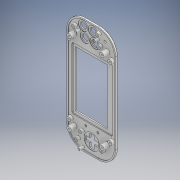
# Autodesk Inventor part: Partie Haute
Saved by Autodesk Inventor 2019 (Build 230136000, 136)
## iProperties
Created: 2018-06-04
Part Number: Partie Haute
Material: Plastique ABS
Document SubType Name: Modeling
Designer: dimercur
Mass: 33.4768 g
Surface Area: 274.719 cm^2
Volume: 31.5819 cm^3
Density: 1.06 g/cm^3
Appearance: Lisse - Blanc
Author: dimercur
Autodesk Inventor part; units mm, degrees
ref_plane "YZ Plane" through (0, 0, 0) normal (1, 0, 0) x (0, 1, 0)
ref_plane "XZ Plane" through (0, 0, 0) normal (0, 1, 0) x (-1, 0, 0)
ref_plane "XY Plane" through (0, 0, 0) normal (0, 0, 1) x (1, 0, 0)
sketch "Esquisse1" plane through (0, 0, 0) normal (0, 1, 0) x (-1, 0, 0)
  line L0 (42.5, 100) -> (-42.5, 100)
  line L1 (-42.5, 100) -> (-42.5, -100)
  line L2 (-42.5, -100) -> (42.5, -100)
  line L3 (42.5, -100) -> (42.5, 100)
  point P0 (0, 0)
  dimension "d0" = 200
  dimension "d1" = 85
  dimension "d2" = 42.5
  dimension "d3" = 100
  constraints: 8 end point, 2 parallel, 1 horizontal, 1 perpendicular
  measures "d0" distance of L2.end L0.start
  measures "d1" distance of L0.start L0.end
  measures "d2" horizontal distance of point (0, 0) L0.start
  measures "d3" vertical distance of point (0, 0) L0.start
extrude "Extrusion1" add sketch "Esquisse1" along normal blind 42
chamfer "Chanfrein1" distance 20 angle 60 1 edges at (0, 0, 100) measured on face at (-14.1667, 14, 100)
chamfer "Chanfrein2" distance 20 angle 60 1 edges at (0, 0, -100) measured on face at (14.1667, 14, -100)
fillet "Congé3" radius 30 4 edges at (-42.5, 31, 100) (42.5, 31, 100) (-42.5, 31, -100) (42.5, 31, -100)
fillet "Congé4" radius 15 14 edges at (0, 0, 65.359) (-33.7132, 14.9269, 91.2132) (-42.5, 1.3397, 67.6795) (33.7132, 14.9269, 91.2132) (42.5, 1.3397, 67.6795) (0, 20, 100) (-42.5, 0, 0) (42.5, 0, 0) (0, 0, -65.359) (33.7132, 14.9269, -91.2132) (42.5, 1.3397, -67.6795) (-33.7132, 14.9269, -91.2132) (-42.5, 1.3397, -67.6795) (0, 20, -100)
shell "Coque1" thickness 2.5 removed faces 1 at (-14.1667, 42, -23.3333)
sketch "Esquisse3" plane through (0, 42, 0) normal (0, 1, 0) x (1, 0, 0)
  arc A0 (42.5, 70) -> (12.5, 100) centre (12.5, 70) ccw projected
  line L0 (12.5, 100) -> (-12.5, 100) projected
  arc A1 (-12.5, 100) -> (-42.5, 70) centre (-12.5, 70) ccw projected
  line L1 (-42.5, 70) -> (-42.5, -70) projected
  arc A2 (-42.5, -70) -> (-12.5, -100) centre (-12.5, -70) ccw projected
  line L2 (-12.5, -100) -> (12.5, -100) projected
  arc A3 (12.5, -100) -> (42.5, -70) centre (12.5, -70) ccw projected
  line L3 (42.5, -70) -> (42.5, 70) projected
  point P0 (0, 0)
extrude "Extrusion2" add sketch "Esquisse3" along normal blind 2.5
sketch "Esquisse4" plane through (0, 44.5, 0) normal (0, 1, 0) x (1, 0, 0)
  line L0 (36.5, 54) -> (-34.5, 54)
  line L1 (-34.5, 54) -> (-34.5, -54)
  line L2 (-34.5, -54) -> (36.5, -54)
  line L3 (36.5, -54) -> (36.5, 54)
  line L4 (27.5, -67.5897) -> (-27.5, -67.5897) projected
  line L5 (42.5, -70) -> (42.5, 70) projected
  line L6 (-42.5, 70) -> (-42.5, -70) projected
  line L7 (12.5, 100) -> (-12.5, 100) projected
  line L8 (-12.5, -100) -> (12.5, -100) projected
  point P0 (0, 0)
  dimension "d19" = 108
  dimension "d20" = 71
  dimension "d21" = 36.5
  dimension "d22" = 54
  dimension "d154" = 85
  dimension "d155" = 46
  constraints: 8 end point, 2 parallel, 1 horizontal, 1 perpendicular
  measures "d19" distance of L2.end L0.start
  measures "d20" distance of L0.start L0.end
  measures "d21" horizontal distance of point (0, 0) L0.start
  measures "d22" vertical distance of point (0, 0) L0.start
  measures "d154" distance between parallel lines of L6 L5
  measures "d155" distance between parallel lines of L8 L2
extrude "Extrusion15" cut sketch "Esquisse4" against normal through all
sketch "Esquisse5" plane through (-40, 15, 61.3397) normal (1, 0, 0) x (0, 0, -1)
  line L0 (-48.6603, 26) -> (171.3397, 26)
  line L1 (171.3397, 26) -> (171.3397, -24)
  line L2 (171.3397, -24) -> (-48.6603, -24)
  line L3 (-48.6603, -24) -> (-48.6603, 26)
  line L4 (-36.1603, 27) -> (-8.6603, 27) projected
  line L5 (-38.6603, 29.5) -> (-38.6603, 13.6603) projected
  line L6 (161.3397, 13.6603) -> (161.3397, 29.5) projected
  point P0 (61.3397, -15)
  dimension "d47" = 1
  dimension "d48" = 220
  dimension "d50" = 200
  dimension "d51" = 10
  dimension "d52" = 50
  constraints: 8 end point, 2 parallel, 1 horizontal, 1 perpendicular
  measures "d47" distance between parallel lines of L4 L0
  measures "d48" distance between parallel lines of L1 L3
  measures "d50" distance between parallel lines of L6 L5
  measures "d51" distance between parallel lines of L5 L3
  measures "d52" distance between parallel lines of L0 L2
extrude "Extrusion4" cut sketch "Esquisse5" along normal through all both and the other way through all
sketch "Esquisse6" plane through (-12.5, 41, -100) normal (0, -1, 0) x (1, 0, 0)
  line L0 (-27.5, 170) -> (-27.5, 30) projected
  arc A0 (-27.5, 30) -> (0, 2.5) centre (0, 30) ccw projected
  line L1 (0, 2.5) -> (25, 2.5) projected
  arc A1 (25, 2.5) -> (52.5, 30) centre (25, 30) ccw projected
  line L2 (52.5, 30) -> (52.5, 170) projected
  arc A2 (52.5, 170) -> (25, 197.5) centre (25, 170) ccw projected
  line L3 (25, 197.5) -> (0, 197.5) projected
  arc A3 (0, 197.5) -> (-27.5, 170) centre (0, 170) ccw projected
  line L4 (-27.75, 30) -> (-27.75, 170)
  arc A4 (0, 197.75) -> (-27.75, 170) centre (0, 170) ccw
  line L5 (0, 197.75) -> (25, 197.75)
  arc A5 (52.75, 170) -> (25, 197.75) centre (25, 170) ccw
  line L6 (52.75, 170) -> (52.75, 30)
  arc A6 (25, 2.25) -> (52.75, 30) centre (25, 30) ccw
  line L7 (25, 2.25) -> (0, 2.25)
  arc A7 (-27.75, 30) -> (0, 2.25) centre (0, 30) ccw
  line L8 (-30, 30) -> (-30, 170) projected
  point P0 (12.5, 100)
  dimension "d55" = 2.5
  dimension "d56" = 0.25
  constraints: 8 end point, 8 point on circle, 4 centre point, 7 other
  measures "d55" distance between parallel lines of L0 L8
  measures "d56" distance between parallel lines of L0 L4
extrude "Extrusion5" cut sketch "Esquisse6" against normal blind 1
sketch "Esquisse7" plane through (0, 42, 0) normal (0, -1, 0) x (1, 0, 0)
  circle A0 centre (-36, -61) radius 3.75
  circle A1 centre (36, -61) radius 3.75
  circle A2 centre (36, 61) radius 3.75
  circle A3 centre (-36, 61) radius 3.75
  point P0 (0, 0)
  dimension "d59" = 7.5
  dimension "d60" = 7.5
  dimension "d61" = 7.5
  dimension "d62" = 7.5
  dimension "d63" = 122
  dimension "d64" = 72
  dimension "d65" = 122
  dimension "d66" = 72
  dimension "d67" = 61
  dimension "d68" = 36
  dimension "d69" = 36
  dimension "d70" = 61
  constraints: 4 centre point
  measures "d59" diameter of A0
  measures "d60" diameter of A1
  measures "d61" diameter of A2
  measures "d62" diameter of A3
  measures "d63" distance of A3.centre A0.centre
  measures "d64" distance of A1.centre A0.centre
  measures "d65" distance of A2.centre A1.centre
  measures "d66" distance of A2.centre A3.centre
  measures "d67" vertical distance of point (0, 0) A0.centre
  measures "d68" horizontal distance of point (0, 0) A3.centre
  measures "d69" horizontal distance of point (0, 0) A0.centre
  measures "d70" vertical distance of point (0, 0) A1.centre
extrude "Extrusion6" add sketch "Esquisse7" along normal blind 4.5
sketch "Esquisse8" plane through (-36, 37.5, -61) normal (0, -1, 0) x (1, 0, 0)
  circle A0 centre (0, 0) radius 1.2
  circle A1 centre (0, 122) radius 1.2
  circle A2 centre (72, 122) radius 1.2
  circle A3 centre (72, 0) radius 1.2
  circle A4 centre (72, 122) radius 3.75 projected
  circle A5 centre (0, 122) radius 3.75 projected
  circle A6 centre (0, 0) radius 3.75 projected
  point P0 (36, 61)
  dimension "d73" = 2.4
  dimension "d74" = 2.4
  dimension "d75" = 2.4
  dimension "d76" = 2.4
  dimension "d77" = 72
  dimension "d78" = 122
  dimension "d79" = 122
  dimension "d80" = 72
  dimension "d81" = 122
  dimension "d82" = 72
  dimension "d83" = 61
  dimension "d84" = 61
  dimension "d85" = 36
  dimension "d86" = 36
  constraints: 4 centre point
  measures "d73" diameter of A0
  measures "d74" diameter of A1
  measures "d75" diameter of A2
  measures "d76" diameter of A3
  measures "d77" distance of A4.centre A5.centre
  measures "d78" distance of A5.centre A6.centre
  measures "d79" distance of A1.centre A0.centre
  measures "d80" distance of A2.centre A1.centre
  measures "d81" distance of A3.centre A2.centre
  measures "d82" distance of A3.centre A0.centre
  measures "d83" vertical distance of point (36, 61) A3.centre
  measures "d84" vertical distance of point (36, 61) A0.centre
  measures "d85" horizontal distance of point (36, 61) A0.centre
  measures "d86" horizontal distance of point (36, 61) A1.centre
extrude "Extrusion7" cut sketch "Esquisse8" against normal blind 5 contours A0 | A1 | A2 | A3
fillet "Congé6" radius 0.5 8 edges at (33.7132, 44.5, -91.2132) (0, 44.5, -100) (-33.7132, 44.5, -91.2132) (-42.5, 44.5, 0) (-33.7132, 44.5, 91.2132) (0, 44.5, 100) (33.7132, 44.5, 91.2132) (42.5, 44.5, 0)
sketch "Esquisse11" plane through (0, 42, 0) normal (0, -1, 0) x (1, 0, 0)
  circle A0 centre (-29.5, -70) radius 4
  circle A1 centre (27.5, -70) radius 4
  circle A2 centre (27.5, 70) radius 4
  circle A3 centre (-29.5, 70) radius 4
  line L0 (-42.5, -70) -> (-42.5, 70) projected
  line L1 (42.5, 70) -> (42.5, -70) projected
  line L2 (12.5, -100) -> (-12.5, -100) projected
  line L3 (-12.5, 100) -> (12.5, 100) projected
  circle A4 centre (-29.5, -70) radius 1.25
  circle A5 centre (27.5, -70) radius 1.25
  circle A6 centre (27.5, 70) radius 1.25
  circle A7 centre (-29.5, 70) radius 1.25
  point P0 (0, 0)
  dimension "d134" = 8
  dimension "d135" = 8
  dimension "d136" = 8
  dimension "d137" = 8
  dimension "d138" = 13
  dimension "d139" = 15
  dimension "d140" = 15
  dimension "d141" = 13
  dimension "d142" = 30
  dimension "d143" = 30
  dimension "d144" = 30
  dimension "d145" = 30
  dimension "d146" = 2.5
  dimension "d147" = 2.5
  dimension "d148" = 2.5
  dimension "d149" = 2.5
  constraints: 8 centre point, 4 coincident
  measures "d134" diameter of A0
  measures "d135" diameter of A1
  measures "d136" diameter of A3
  measures "d137" diameter of A2
  measures "d138" distance from line of L0 A0.centre
  measures "d139" distance from line of L1 A1.centre
  measures "d140" distance from line of L1 A2.centre
  measures "d141" distance from line of L0 A3.centre
  measures "d142" distance from line of A0.centre L2
  measures "d143" distance from line of L2 A1.centre
  measures "d144" distance from line of L3 A2.centre
  measures "d145" distance from line of L3 A3.centre
  measures "d146" diameter of A4
  measures "d147" diameter of A5
  measures "d148" diameter of A7
  measures "d149" diameter of A6
extrude "Extrusion10" add sketch "Esquisse11" along normal blind 10
sketch "Esquisse15" plane through (0, 44.5, 0) normal (0, 1, 0) x (1, 0, 0)
  circle A0 centre (10.5, 62) radius 0.75
  line L0 (-34.5, 54) -> (36.5, 54) projected
  line L1 (42.5, -70) -> (42.5, 70) projected
  circle A1 centre (10.5, 59) radius 0.75
  circle A2 centre (12, 60.5) radius 0.75
  circle A3 centre (9, 60.5) radius 0.75
  circle A4 centre (-10.5, 62) radius 0.75
  circle A5 centre (-10.5, 59) radius 0.75
  circle A6 centre (-9, 60.5) radius 0.75
  circle A7 centre (-12, 60.5) radius 0.75
  point P0 (0, 0)
  dimension "d189" = 1.5
  dimension "d190" = 8
  dimension "d191" = 32
  dimension "d192" = 1.5
  dimension "d193" = 1.5
  dimension "d194" = 1.5
  dimension "d195" = 32
  dimension "d196" = 5
  dimension "d197" = 6.5
  dimension "d198" = 6.5
  dimension "d199" = 3
  dimension "d200" = 3
  dimension "d201" = 30.5
  dimension "d204" = 21
  constraints: 8 centre point, 1 horizontal, 8 other
  measures "d189" diameter of A0
  measures "d190" distance from line of L0 A0.centre
  measures "d191" distance from line of L1 A0.centre
  measures "d192" diameter of A2
  measures "d193" diameter of A1
  measures "d194" diameter of A3
  measures "d195" distance from line of L1 A1.centre
  measures "d196" distance from line of L0 A1.centre
  measures "d197" distance from line of L0 A2.centre
  measures "d198" distance from line of L0 A3.centre
  measures "d199" distance of A0.centre A1.centre
  measures "d200" distance of A3.centre A2.centre
  measures "d201" distance from line of L1 A2.centre
  measures "d204" distance of A0.centre A4.centre
extrude "Extrusion13" cut sketch "Esquisse15" against normal through all
sketch "Esquisse16" plane through (0, 44.5, 0) normal (0, 1, 0) x (1, 0, 0)
  line L0 (40, 57.5) -> (-38, 57.5)
  line L1 (-38, 57.5) -> (-38, -57.5)
  line L2 (-38, -57.5) -> (40, -57.5)
  line L3 (40, -57.5) -> (40, 57.5)
  line L4 (26, 48.5) -> (-30, 48.5)
  line L5 (-30, 48.5) -> (-30, -48.5)
  line L6 (-30, -48.5) -> (26, -48.5)
  line L7 (26, -48.5) -> (26, 48.5)
  line L8 (36.5, 54) -> (36.5, -54) projected
  line L9 (-34.5, 54) -> (36.5, 54) projected
  line L10 (36.5, -54) -> (-34.5, -54) projected
  line L11 (-34.5, -54) -> (-34.5, 54) projected
  point P0 (0, 0)
  dimension "d211" = 97
  dimension "d212" = 48.5
  dimension "d213" = 78
  dimension "d215" = 3.5
  dimension "d217" = 3.5
  dimension "d218" = 3.5
  dimension "d219" = 56
  dimension "d225" = 4.5
  constraints: 16 end point, 4 parallel, 2 horizontal, 2 perpendicular
  measures "d211" distance of L6.end L4.start
  measures "d212" vertical distance of point (0, 0) L4.start
  measures "d213" distance of L0.start L0.end
  measures "d215" distance between parallel lines of L8 L3
  measures "d217" distance between parallel lines of L9 L0
  measures "d218" distance between parallel lines of L10 L2
  measures "d219" distance of L4.start L4.end
  measures "d225" distance between parallel lines of L11 L5
extrude "Extrusion14" add sketch "Esquisse16" along normal blind 1.5 and the other way blind 1 contours L3 L2 L1 L0 | L8 L10 L11 L9
chamfer "Chanfrein4" distance 0.5 angle 45 4 edges at (26, 46, 0) (-2, 46, -48.5) (-2, 46, 48.5) (-30, 46, 0)
fillet "Congé14" radius 8 4 edges at (-38, 45.25, -57.5) (-38, 45.25, 57.5) (40, 45.25, 57.5) (40, 45.25, -57.5)
fillet "Congé15" radius 0.5 16 edges at (37.6569, 44.5, -55.1569) (40, 44.5, 0) (37.6569, 44.5, 55.1569) (1, 44.5, 57.5) (-35.6569, 44.5, 55.1569) (-38, 44.5, 0) (-35.6569, 44.5, -55.1569) (1, 44.5, -57.5) (1, 46, -57.5) (37.6569, 46, -55.1569) (40, 46, 0) (37.6569, 46, 55.1569) (1, 46, 57.5) (-35.6569, 46, 55.1569) (-38, 46, 0) (-35.6569, 46, -55.1569)
fillet "Congé16" radius 3 4 edges at (36.5, 42.75, -54) (-34.5, 42.75, -54) (-34.5, 42.75, 54) (36.5, 42.75, 54)
fillet "Congé17" radius 0.5 8 edges at (35.6213, 43.5, -53.1213) (1, 43.5, -54) (-33.6213, 43.5, -53.1213) (-34.5, 43.5, 0) (-33.6213, 43.5, 53.1213) (1, 43.5, 54) (35.6213, 43.5, 53.1213) (36.5, 43.5, 0)
sketch "Esquisse9" plane through (0, 44.5, 0) normal (0, 1, 0) x (1, 0, 0)
  line L0 (10.75, 83) -> (-10.75, 83)
  line L1 (-10.75, 83) -> (-10.75, 75.5)
  line L2 (-10.75, 75.5) -> (10.75, 75.5)
  line L3 (10.75, 75.5) -> (10.75, 83)
  line L4 (3.75, 90) -> (-3.75, 90)
  line L5 (-3.75, 90) -> (-3.75, 68.5)
  line L6 (-3.75, 68.5) -> (3.75, 68.5)
  line L7 (3.75, 68.5) -> (3.75, 90)
  line L8 (12.5, 100) -> (-12.5, 100) projected
  line L9 (-42.5, 70) -> (-42.5, -70) projected
  line L10 (42.5, -70) -> (42.5, 70) projected
  point P0 (0, 0)
  dimension "d98" = 21.5
  dimension "d99" = 21.5
  dimension "d100" = 7.5
  dimension "d101" = 7.5
  dimension "d102" = 7
  dimension "d103" = 7
  dimension "d104" = 10
  dimension "d105" = 31.75
  dimension "d156" = 85
  constraints: 16 end point, 4 parallel, 2 horizontal, 2 perpendicular
  measures "d98" distance of L6.end L4.start
  measures "d99" distance of L0.start L0.end
  measures "d100" distance of L4.start L4.end
  measures "d101" distance of L2.end L0.start
  measures "d102" distance between parallel lines of L3 L7
  measures "d103" distance from line of L0 L4.start
  measures "d104" distance between parallel lines of L8 L4
  measures "d105" distance between parallel lines of L9 L1
  measures "d156" distance between parallel lines of L9 L10
extrude "Extrusion8" cut sketch "Esquisse9" against normal through all
sketch "Esquisse14" plane through (0, 44.5, 0) normal (0, 1, 0) x (1, 0, 0)
  circle A0 centre (23.25, -83) radius 2.1
  line L0 (-12.5, -100) -> (12.5, -100) projected
  line L1 (42.5, -70) -> (42.5, 70) projected
  circle A1 centre (2, -88) radius 5.5
  circle A2 centre (5, -71.2668) radius 5.5
  circle A3 centre (-12, -71.2668) radius 5.5
  circle A4 centre (-15, -88) radius 5.5
  point P0 (0, 0)
  dimension "d184" = 4.2
  dimension "d185" = 17
  dimension "d186" = 19.25
  dimension "d241" = 11
  dimension "d242" = 11
  dimension "d243" = 11
  dimension "d244" = 11
  dimension "d245" = 17
  dimension "d246" = 17
  dimension "d247" = 28
  dimension "d248" = 28
  dimension "d249" = 2
  dimension "d250" = 12
  dimension "d251" = 12
  dimension "d252" = 5
  constraints: 5 centre point
  measures "d184" diameter of A0
  measures "d185" distance from line of L0 A0.centre
  measures "d186" distance from line of L1 A0.centre
  measures "d241" diameter of A2
  measures "d242" diameter of A1
  measures "d243" diameter of A3
  measures "d244" diameter of A4
  measures "d245" distance of A4.centre A1.centre
  measures "d246" distance of A3.centre A2.centre
  measures "d249" horizontal distance of point (0, 0) A1.centre
  measures "d250" distance from line of L0 A1.centre
  measures "d251" distance from line of L0 A4.centre
  measures "d252" horizontal distance of point (0, 0) A2.centre
extrude "Extrusion12" cut sketch "Esquisse14" against normal through all
sketch "Esquisse12" plane through (0, 42, 0) normal (0, -1, 0) x (1, 0, 0)
  circle A0 centre (21.5, -81.5) radius 3
  circle A1 centre (-22.5, -85) radius 3
  line L0 (12.5, -97.75) -> (-12.5, -97.75) projected
  line L1 (-40.25, -70) -> (-40.25, 70) projected
  line L2 (40.25, 70) -> (40.25, -70) projected
  circle A2 centre (-22.5, -85) radius 1
  circle A3 centre (21.5, -81.5) radius 1
  line L3 (-12.5, 97.75) -> (12.5, 97.75) projected
  circle A4 centre (-16, -70) radius 3
  circle A5 centre (-16, -70) radius 1
  line L4 (-42.5, -70) -> (-42.5, 70) projected
  line L5 (42.5, 70) -> (42.5, -70) projected
  line L6 (12.5, -100) -> (-12.5, -100) projected
  point P0 (0, 0)
  dimension "d157" = 6
  dimension "d158" = 6
  dimension "d166" = 2
  dimension "d167" = 2
  dimension "d288" = 6
  dimension "d289" = 2
  dimension "d306" = 26.5
  dimension "d307" = 20
  dimension "d308" = 21
  dimension "d309" = 18.5
  dimension "d310" = 15
  dimension "d311" = 30
  constraints: 6 centre point, 3 coincident
  measures "d157" diameter of A1
  measures "d158" diameter of A0
  measures "d166" diameter of A2
  measures "d167" diameter of A3
  measures "d288" diameter of A4
  measures "d289" diameter of A5
  measures "d306" distance from line of A4.centre L4
  measures "d307" distance from line of A2.centre L4
  measures "d308" distance from line of A0.centre L5
  measures "d309" distance from line of L6 A0.centre
  measures "d310" distance from line of A1.centre L6
  measures "d311" distance from line of L6 A4.centre
extrude "Extrusion11" add sketch "Esquisse12" along normal blind 4.7
sketch "Esquisse17" plane through (0, 42, 0) normal (0, -1, 0) x (1, 0, 0)
  circle A0 centre (-14.769, -94.179) radius 2
  line L0 (3.75, -90) -> (-3.75, -90) projected
  line L1 (-3.75, -90) -> (-3.75, -83) projected
  point P0 (0, 0)
  dimension "d253" = 4
  dimension "d254" = 4.179
  dimension "d255" = 11.019
  constraints: 1 centre point
  measures "d253" diameter of A0
  measures "d254" distance from line of A0.centre L0
  measures "d255" distance from line of A0.centre L1
extrude "Extrusion16" add sketch "Esquisse17" along normal blind 8
chamfer "Chanfrein5" distance 0.5 angle 45 1 edges at (-16.769, 34, -94.179)
sketch "Esquisse18" plane through (0, 42, 0) normal (0, -1, 0) x (1, 0, 0)
  circle A0 centre (0, -79.25) radius 13.5
  line L0 (3.75, -90) -> (-3.75, -90) projected
  line L1 (-3.75, -68.5) -> (3.75, -68.5) projected
  line L2 (-10.75, -83) -> (-10.75, -75.5) projected
  point P0 (0, 0)
  dimension "d265" = 27
  dimension "d266" = 21.5
  dimension "d267" = 10.75
  dimension "d268" = 10.75
  constraints: 1 centre point
  measures "d265" diameter of A0
  measures "d266" distance between parallel lines of L0 L1
  measures "d267" distance from line of L0 A0.centre
  measures "d268" distance from line of A0.centre L2
extrude "Extrusion17" cut sketch "Esquisse18" against normal blind 0.5
sketch "Esquisse19" plane through (0, 42, 0) normal (0, -1, 0) x (1, 0, 0)
  circle A0 centre (-12, 71.2668) radius 8.25
  circle A1 centre (-15, 88) radius 8.25
  circle A2 centre (2, 88) radius 8.25
  circle A3 centre (5, 71.2668) radius 8.25
  circle A4 centre (-12, 71.2668) radius 5.5 projected
  circle A5 centre (-15, 88) radius 5.5 projected
  circle A6 centre (2, 88) radius 5.5 projected
  circle A7 centre (5, 71.2668) radius 5.5 projected
  point P0 (0, 0)
  dimension "d271" = 16.5
  dimension "d272" = 16.5
  dimension "d273" = 16.5
  dimension "d274" = 16.5
  constraints: 4 centre point, 4 concentric
  measures "d271" diameter of A0
  measures "d272" diameter of A1
  measures "d273" diameter of A2
  measures "d274" diameter of A3
extrude "Extrusion18" cut sketch "Esquisse19" against normal blind 0.5
sketch "Esquisse20" plane through (0, 42, 0) normal (0, -1, 0) x (1, 0, 0)
  circle A0 centre (-21.178, 78.5608) radius 2
  circle A1 centre (11.178, 80.706) radius 2
  circle A2 centre (2, 88) radius 5.5 projected
  circle A3 centre (-12, 71.2668) radius 5.5 projected
  point P0 (0, 0)
  dimension "d277" = 4
  dimension "d278" = 4
  dimension "d279" = 9.178
  dimension "d280" = 7.294
  dimension "d281" = 9.178
  dimension "d282" = 7.294
  constraints: 2 centre point
  measures "d277" diameter of A0
  measures "d278" diameter of A1
  measures "d279" horizontal distance of A1.centre A2.centre
  measures "d280" vertical distance of A1.centre A2.centre
  measures "d281" horizontal distance of A3.centre A0.centre
  measures "d282" vertical distance of A0.centre A3.centre
extrude "Extrusion19" add sketch "Esquisse20" along normal blind 7 contours A0 | A1
chamfer "Chanfrein6" distance 0.5 angle 45 2 edges at (-23.178, 35, 78.5608) (9.178, 35, 80.706)
sketch "Esquisse21" plane through (0, 42, 0) normal (0, -1, 0) x (1, 0, 0)
  circle A0 centre (-27.5, 83) radius 3
  circle A1 centre (-27.5, 83) radius 1
  circle A2 centre (16.5, 73) radius 3
  circle A3 centre (16.5, 73) radius 1
  circle A4 centre (13.5, 91) radius 3
  circle A5 centre (13.5, 91) radius 1
  line L0 (-12.5, 97.75) -> (12.5, 97.75) projected
  line L1 (-40.25, -70) -> (-40.25, 70) projected
  line L2 (-42.5, -70) -> (-42.5, 70) projected
  line L3 (-12.5, 100) -> (12.5, 100) projected
  point P0 (0, 0)
  dimension "d292" = 6
  dimension "d293" = 6
  dimension "d294" = 6
  dimension "d295" = 2
  dimension "d296" = 2
  dimension "d297" = 2
  dimension "d312" = 15
  dimension "d313" = 56
  dimension "d314" = 59
  dimension "d315" = 17
  dimension "d316" = 9
  dimension "d317" = 27
  constraints: 6 centre point, 3 coincident
  measures "d292" diameter of A0
  measures "d293" diameter of A4
  measures "d294" diameter of A2
  measures "d295" diameter of A1
  measures "d296" diameter of A5
  measures "d297" diameter of A3
  measures "d312" distance from line of A0.centre L2
  measures "d313" distance from line of A4.centre L2
  measures "d314" distance from line of A2.centre L2
  measures "d315" distance from line of A0.centre L3
  measures "d316" distance from line of L3 A4.centre
  measures "d317" distance from line of L3 A2.centre
extrude "Extrusion20" add sketch "Esquisse21" along normal blind 4.7
sketch "Esquisse23" plane through (0, 44.5, 0) normal (0, 1, 0) x (1, 0, 0)
  line L0 (12.4498, -76.2889) -> (12.4498, -80.7929) construction
  line L1 (12.4498, -80.7929) -> (8.9498, -80.7929) construction
  line L2 (8.9498, -80.7929) -> (8.9498, -76.2889) construction
  line L3 (8.9498, -76.2889) -> (12.4498, -76.2889) construction
  line L4 (10.9315, -92.2307) -> (10.9315, -96.7078) construction
  line L5 (10.9315, -96.7078) -> (7.4315, -96.7078) construction
  line L6 (7.4315, -96.7078) -> (7.4315, -92.2307) construction
  line L7 (7.4315, -92.2307) -> (10.9315, -92.2307) construction
  line L8 (-4.7066, -76.2889) -> (-4.7066, -81.4265) construction
  line L9 (-4.7066, -81.4265) -> (-8.2066, -81.4265) construction
  line L10 (-8.2066, -81.4265) -> (-8.2066, -76.2889) construction
  line L11 (-8.2066, -76.2889) -> (-4.7066, -76.2889) construction
  line L12 (-7.7432, -92.6861) -> (-7.7432, -97.977) construction
  line L13 (-7.7432, -97.977) -> (-11.2432, -97.977) construction
  line L14 (-11.2432, -97.977) -> (-11.2432, -92.6861) construction
  line L15 (-11.2432, -92.6861) -> (-7.7432, -92.6861) construction
  line L16 (24.2449, -71.0629) -> (24.2449, -77.8436) construction
  line L17 (24.2449, -77.8436) -> (22.1113, -77.8436) construction
  line L18 (22.1113, -77.8436) -> (22.1113, -71.0629) construction
  line L19 (22.1113, -71.0629) -> (24.2449, -71.0629) construction
  line L20 (8.9498, -79.613) -> (8.9498, -78.5976)
  line L21 (8.9498, -78.5976) -> (10.0644, -78.2998)
  line L22 (10.0644, -78.2998) -> (8.9498, -77.2334)
  line L23 (8.9498, -77.2334) -> (8.9498, -76.2605)
  line L24 (8.9498, -76.2605) -> (10.7111, -77.9992)
  line L25 (10.7111, -77.9992) -> (12.4498, -77.4943)
  line L26 (12.4498, -77.4943) -> (12.4498, -78.5125)
  line L27 (12.4498, -78.5125) -> (11.3918, -78.7848)
  line L28 (11.3918, -78.7848) -> (12.4498, -79.7917)
  line L29 (12.4498, -79.7917) -> (12.4498, -80.7646)
  line L30 (12.4498, -80.7646) -> (10.748, -79.0883)
  line L31 (10.748, -79.0883) -> (8.9498, -79.613)
  line L32 (10.9315, -96.6922) -> (8.8922, -94.7919)
  line L33 (8.8922, -94.7919) -> (7.4315, -94.2955)
  line L34 (7.4315, -94.2955) -> (7.4315, -93.4162)
  line L35 (7.4315, -93.4162) -> (8.8497, -93.8984)
  line L36 (8.8497, -93.8984) -> (10.9315, -93.3765)
  line L37 (10.9315, -93.3765) -> (10.9315, -94.3778)
  line L38 (10.9315, -94.3778) -> (9.6835, -94.6387)
  line L39 (9.6835, -94.6387) -> (10.9315, -95.725)
  line L40 (10.9315, -95.725) -> (10.9315, -96.6922)
  spline S0 degree 2 poles (-10.171, -96.2117) (-10.432, -96.1209) (-10.8262, -95.7891) (-10.9567, -95.5792) knots 0 0 0 1 2 2 2
  spline S1 degree 2 poles (-10.9567, -95.5792) (-11.1127, -95.3296) (-11.2432, -94.8134) (-11.2432, -94.4475) knots 0 0 0 1 2 2 2
  line L41 (-11.2432, -94.4475) -> (-11.2432, -93.0492)
  line L42 (-11.2432, -93.0492) -> (-7.7432, -94.2376)
  line L43 (-7.7432, -94.2376) -> (-7.7432, -95.4742)
  spline S2 degree 2 poles (-7.7432, -95.4742) (-7.7432, -95.86) (-7.8027, -96.2344) (-7.8963, -96.3762) knots 0 0 0 1 2 2 2
  spline S3 degree 2 poles (-7.8963, -96.3762) (-7.9956, -96.5322) (-8.3359, -96.6002) (-8.5572, -96.5265) knots 0 0 0 1 2 2 2
  spline S4 degree 2 poles (-8.5572, -96.5265) (-8.8124, -96.4386) (-9.2124, -96.0472) (-9.306, -95.7919) knots 0 0 0 1 2 2 2
  line L44 (-9.306, -95.7919) -> (-9.323, -95.7834)
  spline S5 degree 2 poles (-9.323, -95.7834) (-9.3911, -96.084) (-9.8137, -96.3308) (-10.171, -96.2117) knots 0 0 0 1 2 2 2
  spline S6 degree 2 poles (-10.1569, -95.3069) (-9.9923, -95.3636) (-9.808, -95.2955) (-9.7598, -95.1793) knots 0 0 0 1 2 2 2
  spline S7 degree 2 poles (-9.7598, -95.1793) (-9.7286, -95.1112) (-9.7229, -94.8361) (-9.7229, -94.6007) knots 0 0 0 1 2 2 2
  line L45 (-9.7229, -94.6007) -> (-9.7229, -94.439)
  line L46 (-9.7229, -94.439) -> (-10.605, -94.1383)
  line L47 (-10.605, -94.1383) -> (-10.605, -94.1866)
  spline S8 degree 2 poles (-10.605, -94.1866) (-10.605, -94.5269) (-10.5965, -94.7935) (-10.5369, -94.9495) knots 0 0 0 1 2 2 2
  spline S9 degree 2 poles (-10.5369, -94.9495) (-10.483, -95.0857) (-10.2845, -95.2643) (-10.1569, -95.3069) knots 0 0 0 1 2 2 2
  spline S10 degree 2 poles (-8.7302, -95.5735) (-8.6451, -95.6019) (-8.4664, -95.5763) (-8.4267, -95.4998) knots 0 0 0 1 2 2 2
  spline S11 degree 2 poles (-8.4267, -95.4998) (-8.387, -95.426) (-8.3813, -95.1906) (-8.3813, -94.9552) knots 0 0 0 1 2 2 2
  line L48 (-8.3813, -94.9552) -> (-8.3813, -94.8956)
  line L49 (-8.3813, -94.8956) -> (-9.1244, -94.6432)
  line L50 (-9.1244, -94.6432) -> (-9.1244, -94.7538)
  spline S12 degree 2 poles (-9.1244, -94.7538) (-9.1244, -94.9779) (-9.1159, -95.1622) (-9.0705, -95.2729) knots 0 0 0 1 2 2 2
  spline S13 degree 2 poles (-9.0705, -95.2729) (-9.0195, -95.3948) (-8.8465, -95.5338) (-8.7302, -95.5735) knots 0 0 0 1 2 2 2
  line L51 (-8.2066, -76.2747) -> (-4.7066, -78.6458)
  line L52 (-4.7066, -78.6458) -> (-4.7066, -79.6045)
  line L53 (-4.7066, -79.6045) -> (-8.2066, -79.5988)
  line L54 (-8.2066, -79.5988) -> (-8.2066, -78.6941)
  line L55 (-8.2066, -78.6941) -> (-7.4919, -78.7196)
  line L56 (-7.4919, -78.7196) -> (-7.4919, -77.6163)
  line L57 (-7.4919, -77.6163) -> (-8.2066, -77.1539)
  line L58 (-8.2066, -77.1539) -> (-8.2066, -76.2747)
  line L59 (-6.8565, -78.7423) -> (-5.6993, -78.7763)
  line L60 (-5.6993, -78.7763) -> (-6.8565, -78.0247)
  line L61 (-6.8565, -78.0247) -> (-6.8565, -78.7423)
  line L62 (22.2093, -73.118) -> (22.2093, -72.5069)
  line L63 (22.2093, -72.5069) -> (22.9435, -71.951)
  line L64 (22.9435, -71.951) -> (22.9435, -71.7695)
  line L65 (22.9435, -71.7695) -> (22.2093, -71.7695)
  line L66 (22.2093, -71.7695) -> (22.2093, -71.2703)
  line L67 (22.2093, -71.2703) -> (24.2093, -71.2703)
  line L68 (24.2093, -71.2703) -> (24.2093, -72.0742)
  spline S14 degree 2 poles (24.2093, -72.0742) (24.2093, -72.2411) (24.1672, -72.4875) (24.1023, -72.5928) knots 0 0 0 1 2 2 2
  spline S15 degree 2 poles (24.1023, -72.5928) (24.0343, -72.6998) (23.8219, -72.8262) (23.6599, -72.8262) knots 0 0 0 1 2 2 2
  spline S16 degree 2 poles (23.6599, -72.8262) (23.4313, -72.8262) (23.1445, -72.6188) (23.0602, -72.4453) knots 0 0 0 1 2 2 2
  line L69 (23.0602, -72.4453) -> (22.2093, -73.118)
  spline S17 degree 2 poles (23.5967, -72.3108) (23.6728, -72.3108) (23.7814, -72.2525) (23.8106, -72.186) knots 0 0 0 1 2 2 2
  spline S18 degree 2 poles (23.8106, -72.186) (23.83, -72.139) (23.8414, -72.024) (23.8414, -71.9381) knots 0 0 0 1 2 2 2
  line L70 (23.8414, -71.9381) -> (23.8414, -71.7695)
  line L71 (23.8414, -71.7695) -> (23.3033, -71.7695)
  line L72 (23.3033, -71.7695) -> (23.3033, -71.9137)
  spline S19 degree 2 poles (23.3033, -71.9137) (23.3033, -72.0175) (23.3292, -72.165) (23.3697, -72.2152) knots 0 0 0 1 2 2 2
  spline S20 degree 2 poles (23.3697, -72.2152) (23.4086, -72.2638) (23.5124, -72.3108) (23.5967, -72.3108) knots 0 0 0 1 2 2 2
  line L73 (22.2093, -73.2671) -> (24.2093, -73.2671)
  line L74 (24.2093, -73.2671) -> (24.2093, -74.6188)
  line L75 (24.2093, -74.6188) -> (23.8284, -74.6188)
  line L76 (23.8284, -74.6188) -> (23.8284, -73.7663)
  line L77 (23.8284, -73.7663) -> (23.4767, -73.7663)
  line L78 (23.4767, -73.7663) -> (23.4767, -74.5523)
  line L79 (23.4767, -74.5523) -> (23.0958, -74.5523)
  line L80 (23.0958, -74.5523) -> (23.0958, -73.7663)
  line L81 (23.0958, -73.7663) -> (22.5902, -73.7663)
  line L82 (22.5902, -73.7663) -> (22.5902, -74.6188)
  line L83 (22.5902, -74.6188) -> (22.2093, -74.6188)
  line L84 (22.2093, -74.6188) -> (22.2093, -73.2671)
  spline S21 degree 2 poles (22.1736, -75.5766) (22.1736, -75.3465) (22.2628, -74.9996) (22.3276, -74.8505) knots 0 0 0 1 2 2 2
  line L85 (22.3276, -74.8505) -> (22.8041, -74.8505)
  line L86 (22.8041, -74.8505) -> (22.8041, -74.8959)
  spline S22 degree 2 poles (22.8041, -74.8959) (22.6761, -75.0466) (22.5383, -75.4081) (22.5383, -75.5782) knots 0 0 0 1 2 2 2
  spline S23 degree 2 poles (22.5383, -75.5782) (22.5383, -75.622) (22.5578, -75.763) (22.5772, -75.8052) knots 0 0 0 1 2 2 2
  spline S24 degree 2 poles (22.5772, -75.8052) (22.5999, -75.857) (22.6826, -75.93) (22.749, -75.93) knots 0 0 0 1 2 2 2
  spline S25 degree 2 poles (22.749, -75.93) (22.8252, -75.93) (22.9192, -75.8116) (22.9402, -75.7306) knots 0 0 0 1 2 2 2
  spline S26 degree 2 poles (22.9402, -75.7306) (22.9678, -75.6285) (23.0148, -75.3967) (23.0505, -75.2946) knots 0 0 0 1 2 2 2
  spline S27 degree 2 poles (23.0505, -75.2946) (23.1315, -75.0629) (23.4086, -74.8619) (23.6161, -74.8619) knots 0 0 0 1 2 2 2
  spline S28 degree 2 poles (23.6161, -74.8619) (23.8965, -74.8619) (24.2449, -75.3368) (24.2449, -75.6933) knots 0 0 0 1 2 2 2
  spline S29 degree 2 poles (24.2449, -75.6933) (24.2449, -75.8716) (24.172, -76.2249) (24.1104, -76.3643) knots 0 0 0 1 2 2 2
  line L87 (24.1104, -76.3643) -> (23.6534, -76.3643)
  line L88 (23.6534, -76.3643) -> (23.6534, -76.3206)
  spline S30 degree 2 poles (23.6534, -76.3206) (23.749, -76.2087) (23.8803, -75.8878) (23.8803, -75.7193) knots 0 0 0 1 2 2 2
  spline S31 degree 2 poles (23.8803, -75.7193) (23.8803, -75.6528) (23.8608, -75.5491) (23.8349, -75.4907) knots 0 0 0 1 2 2 2
  spline S32 degree 2 poles (23.8349, -75.4907) (23.8138, -75.4437) (23.7296, -75.3757) (23.6777, -75.3757) knots 0 0 0 1 2 2 2
  spline S33 degree 2 poles (23.6777, -75.3757) (23.5999, -75.3757) (23.5108, -75.4842) (23.4751, -75.6398) knots 0 0 0 1 2 2 2
  spline S34 degree 2 poles (23.4751, -75.6398) (23.4524, -75.7403) (23.4086, -75.9267) (23.3714, -76.0337) knots 0 0 0 1 2 2 2
  spline S35 degree 2 poles (23.3714, -76.0337) (23.2952, -76.2411) (23.0424, -76.4437) (22.8349, -76.4437) knots 0 0 0 1 2 2 2
  spline S36 degree 2 poles (22.8349, -76.4437) (22.5367, -76.4437) (22.1736, -75.9753) (22.1736, -75.5766) knots 0 0 0 1 2 2 2
  line L89 (22.2093, -76.7014) -> (24.2093, -76.7014)
  line L90 (24.2093, -76.7014) -> (24.2093, -78.0531)
  line L91 (24.2093, -78.0531) -> (23.8284, -78.0531)
  line L92 (23.8284, -78.0531) -> (23.8284, -77.2006)
  line L93 (23.8284, -77.2006) -> (23.4767, -77.2006)
  line L94 (23.4767, -77.2006) -> (23.4767, -77.9867)
  line L95 (23.4767, -77.9867) -> (23.0958, -77.9867)
  line L96 (23.0958, -77.9867) -> (23.0958, -77.2006)
  line L97 (23.0958, -77.2006) -> (22.5902, -77.2006)
  line L98 (22.5902, -77.2006) -> (22.5902, -78.0531)
  line L99 (22.5902, -78.0531) -> (22.2093, -78.0531)
  line L100 (22.2093, -78.0531) -> (22.2093, -76.7014)
  line L101 (22.2093, -78.7776) -> (23.8284, -78.7776)
  line L102 (23.8284, -78.7776) -> (23.8284, -78.186)
  line L103 (23.8284, -78.186) -> (24.2093, -78.186)
  line L104 (24.2093, -78.186) -> (24.2093, -79.8716)
  line L105 (24.2093, -79.8716) -> (23.8284, -79.8716)
  line L106 (23.8284, -79.8716) -> (23.8284, -79.28)
  line L107 (23.8284, -79.28) -> (22.2093, -79.28)
  line L108 (22.2093, -79.28) -> (22.2093, -78.7776)
  point P0 (0, 0)
  constraints: 10 other
emboss "Gravure1" sketch "Esquisse23" operation cut depth 0.5 direction (0, -1, 0)
sketch "Esquisse24" plane through (0, 46, 0) normal (0, 1, 0) x (1, 0, 0)
  line L0 (38, 31) -> (38, -31) construction
  line L1 (38, -31) -> (26.613, -31) construction
  line L2 (26.613, -31) -> (26.613, 31) construction
  line L3 (26.613, 31) -> (38, 31) construction
  line L4 (39.5, 49.5) -> (39.5, -49.5) projected
  line L5 (29.4106, 26.9846) -> (36.4106, 22.2423)
  line L6 (36.4106, 22.2423) -> (36.4106, 20.325)
  line L7 (36.4106, 20.325) -> (29.4106, 20.3363)
  line L8 (29.4106, 20.3363) -> (29.4106, 22.1459)
  line L9 (29.4106, 22.1459) -> (30.8401, 22.0948)
  line L10 (30.8401, 22.0948) -> (30.8401, 24.3015)
  line L11 (30.8401, 24.3015) -> (29.4106, 25.2261)
  line L12 (29.4106, 25.2261) -> (29.4106, 26.9846)
  line L13 (32.1108, 22.0494) -> (34.4252, 21.9814)
  line L14 (34.4252, 21.9814) -> (32.1108, 23.4846)
  line L15 (32.1108, 23.4846) -> (32.1108, 22.0494)
  line L16 (29.4106, 13.1718) -> (29.4106, 15.3104)
  line L17 (29.4106, 15.3104) -> (31.9803, 16.3825)
  line L18 (31.9803, 16.3825) -> (31.9803, 17.0178)
  line L19 (31.9803, 17.0178) -> (29.4106, 17.8914)
  line L20 (29.4106, 17.8914) -> (29.4106, 19.6386)
  line L21 (29.4106, 19.6386) -> (36.4106, 17.2618)
  line L22 (36.4106, 17.2618) -> (36.4106, 14.4425)
  spline S0 degree 2 poles (36.4106, 14.4425) (36.4106, 13.8639) (36.2631, 13.047) (36.0362, 12.7577) knots 0 0 0 1 2 2 2
  spline S1 degree 2 poles (36.0362, 12.7577) (35.798, 12.4627) (35.0549, 12.2755) (34.4876, 12.4684) knots 0 0 0 1 2 2 2
  spline S2 degree 2 poles (34.4876, 12.4684) (33.6878, 12.7407) (32.6837, 13.8071) (32.3888, 14.5105) knots 0 0 0 1 2 2 2
  line L23 (32.3888, 14.5105) -> (29.4106, 13.1718)
  spline S3 degree 2 poles (34.2664, 14.346) (34.533, 14.2553) (34.9131, 14.329) (35.0152, 14.5276) knots 0 0 0 1 2 2 2
  spline S4 degree 2 poles (35.0152, 14.5276) (35.0832, 14.6694) (35.123, 15.0608) (35.123, 15.3614) knots 0 0 0 1 2 2 2
  line L24 (35.123, 15.3614) -> (35.123, 15.9514)
  line L25 (35.123, 15.9514) -> (33.2396, 16.5924)
  line L26 (33.2396, 16.5924) -> (33.2396, 16.0875)
  spline S5 degree 2 poles (33.2396, 16.0875) (33.2396, 15.7188) (33.3304, 15.1799) (33.4722, 14.9473) knots 0 0 0 1 2 2 2
  spline S6 degree 2 poles (33.4722, 14.9473) (33.6084, 14.7374) (33.9714, 14.4481) (34.2664, 14.346) knots 0 0 0 1 2 2 2
  line L27 (29.4106, 5.5024) -> (29.4106, 7.2496)
  line L28 (29.4106, 7.2496) -> (34.0508, 5.6726)
  line L29 (34.0508, 5.6726) -> (31.0557, 7.9643)
  line L30 (31.0557, 7.9643) -> (31.0557, 9.1613)
  line L31 (31.0557, 9.1613) -> (34.0508, 9.4165)
  line L32 (34.0508, 9.4165) -> (29.4106, 10.9935)
  line L33 (29.4106, 10.9935) -> (29.4106, 12.6499)
  line L34 (29.4106, 12.6499) -> (36.4106, 10.2731)
  line L35 (36.4106, 10.2731) -> (36.4106, 8.2423)
  line L36 (36.4106, 8.2423) -> (32.956, 7.8679)
  line L37 (32.956, 7.8679) -> (36.4106, 5.1451)
  line L38 (36.4106, 5.1451) -> (36.4106, 3.1256)
  line L39 (36.4106, 3.1256) -> (29.4106, 5.5024)
  line L40 (36.7226, -5.2188) -> (27.8904, 0.5673)
  line L41 (27.8904, 0.5673) -> (27.8904, 1.9173)
  line L42 (27.8904, 1.9173) -> (36.7226, -3.863)
  line L43 (36.7226, -3.863) -> (36.7226, -5.2188)
  line L44 (29.4106, -6.3874) -> (36.4106, -11.1297)
  line L45 (36.4106, -11.1297) -> (36.4106, -13.047)
  line L46 (36.4106, -13.047) -> (29.4106, -13.0357)
  line L47 (29.4106, -13.0357) -> (29.4106, -11.2261)
  line L48 (29.4106, -11.2261) -> (30.8401, -11.2771)
  line L49 (30.8401, -11.2771) -> (30.8401, -9.0705)
  line L50 (30.8401, -9.0705) -> (29.4106, -8.1459)
  line L51 (29.4106, -8.1459) -> (29.4106, -6.3874)
  line L52 (32.1108, -11.3225) -> (34.4252, -11.3906)
  line L53 (34.4252, -11.3906) -> (32.1108, -9.8874)
  line L54 (32.1108, -9.8874) -> (32.1108, -11.3225)
  spline S7 degree 2 poles (32.905, -21.1645) (31.9236, -20.8355) (30.3807, -19.4514) (29.9666, -18.6629) knots 0 0 0 1 2 2 2
  spline S8 degree 2 poles (29.9666, -18.6629) (29.6148, -17.9935) (29.4106, -16.6434) (29.4106, -15.923) knots 0 0 0 1 2 2 2
  line L55 (29.4106, -15.923) -> (29.4106, -13.7334)
  line L56 (29.4106, -13.7334) -> (36.4106, -16.1102)
  line L57 (36.4106, -16.1102) -> (36.4106, -18.2828)
  spline S9 degree 2 poles (36.4106, -18.2828) (36.4106, -19.0203) (36.2234, -20.2399) (35.8604, -20.6823) knots 0 0 0 1 2 2 2
  spline S10 degree 2 poles (35.8604, -20.6823) (35.4179, -21.2212) (33.9204, -21.5105) (32.905, -21.1645) knots 0 0 0 1 2 2 2
  spline S11 degree 2 poles (32.9163, -19.3663) (33.6084, -19.6045) (34.5954, -19.4627) (34.8734, -19.0656) knots 0 0 0 1 2 2 2
  spline S12 degree 2 poles (34.8734, -19.0656) (35.0662, -18.7763) (35.1059, -18.0049) (35.1059, -17.4603) knots 0 0 0 1 2 2 2
  line L58 (35.1059, -17.4603) -> (35.1059, -17.4263)
  line L59 (35.1059, -17.4263) -> (30.721, -15.94)
  line L60 (30.721, -15.94) -> (30.721, -15.9684)
  spline S13 degree 2 poles (30.721, -15.9684) (30.721, -16.5583) (30.7607, -17.3865) (30.9933, -17.829) knots 0 0 0 1 2 2 2
  spline S14 degree 2 poles (30.9933, -17.829) (31.2656, -18.3566) (32.2242, -19.1337) (32.9163, -19.3663) knots 0 0 0 1 2 2 2
  line L61 (29.4106, -20.2682) -> (36.4106, -25.0105)
  line L62 (36.4106, -25.0105) -> (36.4106, -26.9279)
  line L63 (36.4106, -26.9279) -> (29.4106, -26.9165)
  line L64 (29.4106, -26.9165) -> (29.4106, -25.107)
  line L65 (29.4106, -25.107) -> (30.8401, -25.158)
  line L66 (30.8401, -25.158) -> (30.8401, -22.9514)
  line L67 (30.8401, -22.9514) -> (29.4106, -22.0267)
  line L68 (29.4106, -22.0267) -> (29.4106, -20.2682)
  line L69 (32.1108, -25.2034) -> (34.4252, -25.2715)
  line L70 (34.4252, -25.2715) -> (32.1108, -23.7682)
  line L71 (32.1108, -23.7682) -> (32.1108, -25.2034)
  point P0 (0, 0)
  dimension "d324" = 31
  dimension "d325" = 62
  dimension "d326" = 1.5
  constraints: 2 other
  measures "d324" vertical distance of point (0, 0) L0.start
  measures "d325" distance of L0.start L0.end
  measures "d326" distance from line of L4 L0.start
emboss "Gravure2" sketch "Esquisse24" operation cut depth 0.5 direction (0, -1, 0)
equation "\"d2\" = 0.5 * d1"
equation "\"d3\" = 0.5 * d0"
equation "\"d22\" = 0.5 * d19"
equation "\"d51\" = -0.5 * d50 + 0.5 * d48"
equation "\"d60\" = d59"
equation "\"d61\" = d59"
equation "\"d62\" = d59"
equation "\"d65\" = d63"
equation "\"d66\" = d64"
equation "\"d67\" = 0.5 * d63"
equation "\"d68\" = 0.5 * d66"
equation "\"d69\" = 0.5 * d64"
equation "\"d70\" = 0.5 * d63"
equation "\"d74\" = d73"
equation "\"d75\" = d73"
equation "\"d76\" = d73"
equation "\"d79\" = d78"
equation "\"d80\" = d77"
equation "\"d81\" = d78"
equation "\"d82\" = d77"
equation "\"d83\" = 0.5 * d78"
equation "\"d84\" = 0.5 * d78"
equation "\"d85\" = 0.5 * d77"
equation "\"d86\" = 0.5 * d77"
equation "\"d135\" = d134"
equation "\"d136\" = d134"
equation "\"d137\" = d134"
equation "\"d140\" = d139"
equation "\"d141\" = d138"
equation "\"d143\" = d142"
equation "\"d144\" = d143"
equation "\"d145\" = d142"
equation "\"d147\" = d146"
equation "\"d148\" = d146"
equation "\"d149\" = d146"
equation "\"d192\" = d189"
equation "\"d193\" = d189"
equation "\"d194\" = d189"
equation "\"d198\" = d197"
equation "\"d200\" = d199"
equation "\"d212\" = 0.5 * d211"
equation "\"d217\" = d215"
equation "\"d218\" = d215"
equation "\"d99\" = d98"
equation "\"d101\" = d100"
equation "\"d102\" = -0.5 * d100 + 0.5 * d98"
equation "\"d103\" = -0.5 * d100 + 0.5 * d98"
equation "\"d105\" = 0.5 * d156 - 0.5 * d98"
equation "\"d158\" = d157"
equation "\"d167\" = d166"
